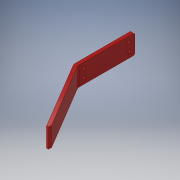
# Autodesk Inventor part: XZ chain Support top
Saved by Autodesk Inventor 2018.2 (Build 222227000, 227)
## iProperties
Created: 2018-01-22
Part Number: XZ chain Support top
Material: Generic
Document SubType Name: Modeling
Designer: torba
Density: 1 g/cm^3
Appearance: Red
Mass: 63.8145 g
Surface Area: 244.205 cm^2
Volume: 63.8145 cm^3
Author: torba
Autodesk Inventor part; units mm, degrees
ref_plane "YZ Plane" through (0, 0, 0) normal (1, 0, 0) x (0, 1, 0)
ref_plane "XZ Plane" through (0, 0, 0) normal (0, 1, 0) x (-1, 0, 0)
ref_plane "XY Plane" through (0, 0, 0) normal (0, 0, 1) x (1, 0, 0)
sketch "Sketch1" plane through (0, 0, 0) normal (0, 1, 0) x (-1, 0, 0)
  line L0 (83.185, 191.7556) -> (83.185, 198.1056)
  line L1 (159.385, -48.7444) -> (165.735, -48.7444)
  line L2 (165.735, -48.7444) -> (165.735, 65.7049)
  line L3 (88.6391, 195.0075) -> (165.735, 65.7049)
  line L4 (88.6391, 195.0075) -> (86.7919, 198.1056)
  line L5 (83.185, 198.1056) -> (86.7919, 198.1056)
  line L6 (159.385, 63.9556) -> (159.385, -48.7444)
  line L7 (165.735, 65.7049) -> (159.385, 63.9556)
  line L8 (83.185, 191.7556) -> (159.385, 63.9556)
  line L9 (162.56, -48.7444) -> (162.56, 64.8303)
  line L10 (162.56, 64.8303) -> (83.185, 198.1056)
  point P0 (0, 0)
  point P1 (0, 0)
  point P2 (0, 0)
  point P3 (0, 0)
  dimension "d22" = 6.35
  dimension "d25" = 6.35
  dimension "d26" = 3.6069
  dimension "d28" = 77.0959
  dimension "d29" = 114.4494
  constraints: 22 end point, 2 horizontal, 2 midpoint, 2 vertical, 1 perpendicular
  measures "d22" distance of L1.start L1.end
  measures "d25" distance of L0.start L0.end
  measures "d26" distance of L0.end L4.end
  measures "d28" horizontal distance of L3.start L2.end
  measures "d29" distance of L1.end L2.end
extrude "Extrusion3" add sketch "Sketch1" along normal blind 38.1
fillet "Fillet2" radius 12.7 2 edges at (-165.735, 19.05, 65.7049) (-159.385, 19.05, 63.9556)
fillet "Fillet3" radius 3.175 2 edges at (-162.56, 38.1, -48.7444) (-162.56, 0, -48.7444)
sketch "Sketch3" plane through (-165.735, 0, 62.2062) normal (-1, 0, 0) x (0, 0, 1)
  circle A0 centre (-9.6006, 11.05) radius 3
  circle A1 centre (-9.6006, 27.05) radius 3
  circle A2 centre (-99.6006, 11.05) radius 3
  circle A3 centre (-99.6006, 27.05) radius 3
  line L0 (-107.7756, 0) -> (0, 0) projected
  line L1 (-99.6006, 27.05) -> (-99.6006, 11.05) construction
  line L2 (-1.7494, 0) -> (-107.7756, 0) projected
  line L3 (-99.6006, 0) -> (-99.6006, 38.1) construction
  line L4 (-1.7494, 38.1) -> (-107.7756, 38.1) projected
  point P0 (-62.2062, 0)
  point P1 (-99.6006, 19.05)
  point P2 (-99.6006, 19.05)
  constraints: 4 centre point, 4 end point, 2 midpoint, 2 point on line, 1 vertical
extrude "Extrusion4" cut sketch "Sketch3" against normal through all
body "Solid2"
